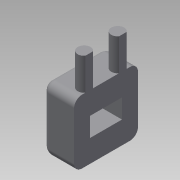
# Autodesk Inventor part: pig_butt
Saved by Autodesk Inventor 2015 (Build 190159000, 159)
## iProperties
Created: 2016-04-29
Part Number: pig_butt
Material: Generic
Document SubType Name: Modeling
Designer: Luke Good
Density: 1 g/cm^3
Appearance: Default
Author: Luke Good
Autodesk Inventor part; units mm, degrees
ref_plane "YZ Plane" through (0, 0, 0) normal (1, 0, 0) x (0, 1, 0)
ref_plane "XZ Plane" through (0, 0, 0) normal (0, 1, 0) x (-1, 0, 0)
ref_plane "XY Plane" through (0, 0, 0) normal (0, 0, 1) x (1, 0, 0)
sketch "Sketch1" plane through (0, 0, 0) normal (0, 0, 1) x (1, 0, 0)
  line L0 (6.35, -12.6955) -> (-3.175, -12.6955)
  line L1 (-6.35, -9.5205) -> (-6.35, 9.5205)
  line L2 (-3.175, 12.6955) -> (6.35, 12.6955)
  line L3 (6.35, 12.6955) -> (6.35, -12.6955)
  line L4 (6.35, -12.6955) -> (-6.35, 12.6955) construction
  line L5 (-6.35, -12.6955) -> (6.35, 12.6955) construction
  arc A0 (-3.175, 12.6955) -> (-6.35, 9.5205) centre (-3.175, 9.5205) ccw
  arc A1 (-6.35, -9.5205) -> (-3.175, -12.6955) centre (-3.175, -9.5205) ccw
  point P0 (0, 0)
  dimension "d0" = 12.7
  dimension "d1" = 3.175
  constraints: 12 end point, 4 point on circle, 4 point on line, 4 tangent, 2 centre point, 2 midpoint, 2 parallel, 1 equal radius, 1 horizontal, 1 perpendicular
  measures "d0" distance of L4.end L2.end
  measures "d1" radius of A0
extrude "Extrusion1" add sketch "Sketch1" along normal blind 25.4
fillet "Fillet1" radius 3.175 10 edges at (-6.35, 0, 25.4) (-5.4201, -11.7656, 25.4) (1.5875, -12.6955, 25.4) (1.5875, 12.6955, 25.4) (-5.4201, 11.7656, 25.4) (-5.4201, 11.7656, 0) (1.5875, 12.6955, 0) (-5.4201, -11.7656, 0) (1.5875, -12.6955, 0) (-6.35, 0, 0)
sketch "Sketch2" plane through (-3.175, 12.6955, 3.175) normal (0, 1, 0) x (1, 0, 0)
  arc A0 (9.525, -14.6582) -> (9.525, -17.7537) centre (7.511, -16.206) ccw
  line L0 (0, 0) -> (0, -19.05) projected
  line L1 (9.525, 0) -> (9.525, -19.05) projected
  arc A1 (9.525, -1.2963) -> (9.525, -4.3918) centre (7.511, -2.844) ccw
  line L2 (9.525, -1.2963) -> (9.525, -4.3918)
  line L3 (9.525, -14.6582) -> (9.525, -17.7537)
  point P0 (3.175, 3.175)
  dimension "d5" = 5.08
  constraints: 4 end point, 4 point on circle, 4 point on line, 2 centre point
  measures "d5" diameter of A0
extrude "Extrusion2" add sketch "Sketch2" along normal blind 12.7
sketch "Sketch3" plane through (-6.35, -9.5205, 3.175) normal (-1, 0, 0) x (0, 0, 1)
  line L0 (4.445, 6.9805) -> (9.525, 9.5205) construction
  line L1 (9.525, 9.5205) -> (4.445, 11.5525) construction
  line L2 (3.175, 6.9805) -> (9.525, 9.5205) construction
  line L3 (9.525, 9.5205) -> (5.2917, 12.0605) construction
  line L4 (5.2917, 6.9805) -> (13.7583, 12.0605) construction
  line L5 (3.175, 13.3305) -> (3.175, 5.7105)
  line L6 (15.875, 5.7105) -> (15.875, 13.3305)
  line L7 (14.9679, 13.3305) -> (3.175, 5.0755) construction
  line L8 (4.0821, 13.3305) -> (14.9679, 5.7105) construction
  line L9 (3.175, 5.0755) -> (3.175, 5.7105)
  line L10 (15.875, 5.7105) -> (15.875, 13.3305)
  line L11 (3.175, 13.3305) -> (3.175, 5.7105)
  line L12 (3.175, 13.3305) -> (15.875, 13.3305)
  line L13 (3.175, 5.7105) -> (15.875, 5.7105)
  point P0 (-3.175, 9.5205)
  point P1 (9.525, 9.5205)
  constraints: 28 end point, 8 point on line, 3 midpoint, 2 equal length, 1 perpendicular
extrude "Extrusion3" cut sketch "Sketch3" against normal blind 12.7
body "Solid1"
